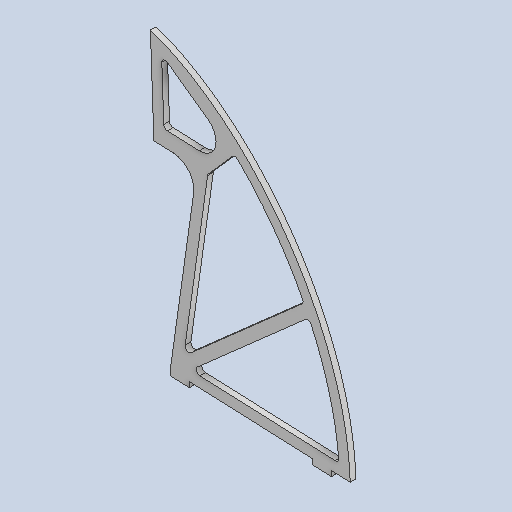
# Autodesk Inventor part: aux_nose_side
Saved by Autodesk Inventor 2022 (Build 260153000, 153)
## iProperties
Created: 2021-04-25
Part Number: aux_nose_side
Material: Generic
Document SubType Name: Modeling
Designer: kardo
Density: 1 g/cm^3
Appearance: Default
Mass: 3.39885 g
Surface Area: 48.7816 cm^2
Volume: 3.39885 cm^3
Author: kardo
Autodesk Inventor part; units mm, degrees
ref_plane "YZ Plane" through (0, 0, 0) normal (1, 0, 0) x (0, 1, 0)
ref_plane "XZ Plane" through (0, 0, 0) normal (0, 1, 0) x (-1, 0, 0)
ref_plane "XY Plane" through (0, 0, 0) normal (0, 0, 1) x (1, 0, 0)
derived "frame_outline.ipt"
sketch "aux_nose_side" plane through (81, 0, 28.1718) normal (0.0377663, 0.0348746, -0.9986779) x (0, 0.9993908, 0.0348995)
  line L0 (128.7776, 3.0021) -> (235.4965, 2.9535)
  line L1 (128.6834, 74.4231) -> (128.7776, 3.0021)
  line L2 (128.9392, -119.5453) -> (128.6076, 131.935)
  spline S0 degree 3 poles (128.6824, 75.2231) (178.453, 75.2888) (227.2802, 39.4794) (237.1445, 0) knots 0 0 0 0 1 1 1 1
  spline S1 degree 3 poles (128.6834, 74.4231) (132.6879, 74.4284) (140.6866, 73.9709) (150.5583, 72.3128) (160.2588, 69.9034) (167.8516, 67.4004) (177.0566, 63.6161) (184.1611, 60.0898) (192.6408, 55.123) (199.0732, 50.7282) (206.598, 44.7729) (212.1746, 39.6654) (218.5154, 32.9174) (223.0538, 27.2545) (227.9834, 19.911) (232.1324, 12.3358) (234.54, 6.0988) (235.4965, 2.9535) knots 0 0 0 0 0.081085 0.162171 0.202713 0.283799 0.324342 0.405427 0.44597 0.527055 0.567598 0.648683 0.689226 0.770311 0.810854 0.891939 0.973025 0.973025 0.973025 0.973025
  point P0 (-0.9832, -82.0055)
  point P1 (235.8467, 2.9533)
  point P2 (204.0556, 3.0021)
extrude "plate" add sketch "aux_nose_side" along normal blind 2
sketch "Sketch2" plane through (84, 128.6952, 32.7794) normal (-0.0377663, -0.0348746, 0.9986779) x (0.9992865, -0.0008625, 0.0377592)
  line L0 (71.4209, -0.1267) -> (0, 0) projected
  line L1 (71.4209, -0.1267) -> (0, 0) projected
  line L2 (57.1367, -0.1014) -> (57.1332, -2.1014)
  line L3 (57.1332, -2.1014) -> (64.2753, -2.1141)
  line L4 (64.2753, -2.1141) -> (64.2788, -0.1141)
  line L5 (3.571, -0.0063) -> (3.5675, -2.0063)
  line L6 (3.5675, -2.0063) -> (10.7096, -2.019)
  line L7 (10.7096, -2.019) -> (10.7131, -0.019)
  point P0 (-85.0668, -129.722)
  point P1 (64.2788, -0.1141)
  point P2 (57.1367, -0.1014)
  point P3 (10.7131, -0.019)
  point P4 (3.571, -0.0063)
  dimension "d28" = 71.421
  dimension "d29" = 7.1421
  dimension "d30" = 7.1421
  dimension "d31" = 2
  dimension "d32" = 3.5711
  dimension "d33" = 7.1421
  constraints: 12 end point, 4 perpendicular, 4 point on line, 2 parallel, 1 collinear
  measures "d28" distance of L0.start L0.end
  measures "d29" distance of L5.end L6.end
  measures "d30" distance of L2.end L3.end
  measures "d31" distance of L2.start L2.end
  measures "d32" distance of L5.start L0.end
  measures "d33" distance of L0.start L4.end
extrude "fins_break_plane" add sketch "Sketch2" against normal up to surface (2 mm away)
sketch "Sketch3" plane through (84, 128.6952, 32.7794) normal (-0.0377663, -0.0348746, 0.9986779) x (0.9992865, -0.0008625, 0.0377592)
  line L0 (10.7096, -2.019) -> (10.7131, -0.019) projected
  line L1 (57.1367, -0.1014) -> (57.1332, -2.1014) projected
  line L2 (0, 0) -> (0, 106.7189) projected
  spline S0 degree 3 poles (0, 106.7189) (3.1449, 105.7609) (9.3807, 103.3505) (16.954, 99.198) (24.2953, 94.2651) (29.9562, 89.7242) (36.7013, 83.3803) (41.8062, 77.8013) (47.758, 70.2738) (52.1499, 63.8394) (57.1129, 55.3575) (60.6359, 48.2513) (64.4161, 39.0446) (66.9157, 31.4506) (69.3206, 21.7491) (70.9741, 11.8766) (71.428, 3.8777) (71.4209, -0.1267) knots 0 0 0 0 0.083333 0.166667 0.208333 0.291667 0.333333 0.416667 0.458333 0.541667 0.583333 0.666667 0.708333 0.791667 0.833333 0.916667 1 1 1 1
  line L3 (3.571, -0.0063) -> (3.5675, -2.0063) projected
  line L4 (3.571, -0.0063) -> (14.7068, 62.4987)
  arc A0 (14.7068, 62.4987) -> (7.3534, 71.278) centre (7.3534, 63.8088) ccw
  line L5 (10.7131, -0.019) -> (10.3569, -2.0184) construction
  line L6 (3.5675, -2.0063) -> (10.7096, -2.019) projected
  line L7 (4, 77.278) -> (4, 101.0748)
  line L8 (8.3452, 3.9852) -> (67.3476, 3.8805)
  line L9 (71.4209, -0.1267) -> (64.2788, -0.1141) projected
  line L10 (7.3534, 71.278) -> (0, 71.278)
  line L11 (20.3339, 71.278) -> (8.3452, 3.9852)
  line L12 (3.571, -0.0063) -> (0, 0) projected
  line L13 (57.1367, -0.1014) -> (10.7131, -0.019) projected
  line L14 (8.9123, 7.1685) -> (55.7843, 48.9138)
  line L15 (11.3463, 3.9799) -> (57.5385, 45.1197)
  line L16 (17.3398, 77.278) -> (4, 77.278)
  arc A1 (17.3398, 77.278) -> (21.0802, 89.2615) centre (17.3398, 83.8535) ccw
  line L17 (21.0802, 89.2615) -> (4, 101.0748)
  line L18 (21.0802, 89.2615) -> (22.1137, 90.7559) construction
  line L19 (8.3452, 3.9852) -> (56.6752, 47.0291) construction
  line L20 (22.2644, 79.4962) -> (17.3398, 83.8535) construction
  line L21 (22.2644, 79.4962) -> (25.2601, 76.8456) construction
  line L22 (56.6752, 47.0291) -> (67.3476, 3.8805) construction
  line L23 (20.3339, 71.278) -> (30.952, 83.2785)
  line L24 (56.6752, 47.0291) -> (30.952, 83.2785) construction
  line L25 (0, 62.4987) -> (14.7068, 62.4987) construction
  line L26 (7.3534, 71.278) -> (7.3534, 62.4987) construction
  line L27 (0, 71.278) -> (0, 73.2783)
  line L28 (0, 73.2783) -> (0.0343, 75.278)
  line L29 (0.0343, 75.278) -> (0, 77.278)
  line L30 (0, 77.278) -> (4, 77.278)
  spline S1 degree 5 poles (4, 101.0748) (10.439, 98.5043) (16.5509, 95.1144) (22.262, 91.1174) (34.4968, 80.8283) (44.6435, 68.432) (49.7053, 60.9368) (58.1785, 45.5925) (63.8074, 29.0036) (65.8171, 20.7435) (67.0242, 12.3289) (67.3477, 3.8805) knots 0 0 0 0 0 0 0.284299 0.284299 0.284299 0.653322 0.653322 0.653322 1 1 1 1 1 1
  point P0 (-85.0668, -129.722)
  point P1 (64.2788, -0.1141)
  dimension "d41" = 4
  dimension "d12" = 106.7189
  dimension "d14" = 4
  dimension "d15" = 4
  dimension "d18" = 170
  dimension "d25" = 4
  dimension "d35" = 4
  dimension "d38" = 5
  dimension "d39" = 6
  dimension "d40" = 4
  dimension "d50" = 2
  constraints: 46 end point, 10 point on line, 5 parallel, 5 perpendicular, 5 point on circle, 4 tangent, 2 centre point, 2 collinear, 2 equal length, 1 midpoint, 1 vertical, 12 other
  measures "d12" distance of L2.start L2.end
  measures "d14" distance of the line from the sketch origin of L8
  measures "d15" distance between parallel lines of L2 L7
  measures "d18" angle of L5 L0
  measures "d25" distance between parallel lines of L14 L15
  measures "d35" distance between parallel lines of L4 L11
  measures "d39" distance between parallel lines of L10 L16
  measures "d40" distance of L20.start L21.end
  measures "d50" distance of L27.end L28.end
extrude "Extrusion4" cut sketch "Sketch3" against normal through all contours L2 L10 A0 L4 L12 | L7 L17 A1 L16 | L15 S1 L8
sketch "Sketch4" plane through (127.8536, 187.3715, 36.4868) normal (-0.0377663, -0.0348746, 0.9986779) x (0.9992857, -0.002636, 0.0376972)
  line L0 (-32.4682, -54.8278) -> (13.6509, -13.606) projected
  line L1 (-29.2116, 3.697) -> (-40.2363, -58.8278) projected
  arc A0 (-26.6048, 18.4808) -> (-22.8856, 30.471) centre (-26.6164, 25.0564) ccw projected
  line L2 (-34.9079, -51.6434) -> (11.89, -9.815)
  line L3 (-13.0033, 24.5055) -> (-23.6001, 12.4862)
  line L4 (-23.6001, 12.4862) -> (-34.9079, -51.6434)
  arc A1 (-26.6048, 18.4808) -> (-22.8856, 30.471) centre (-26.6164, 25.0564) ccw projected
  line L5 (-18.6837, 18.0625) -> (-26.6164, 25.0564) construction
  line L6 (-43.9339, 12.4501) -> (-36.5805, 12.4631) projected
  arc A2 (11.89, -9.815) -> (-13.0033, 24.5055) centre (-95.4946, -61.5148) ccw
  point P0 (-128.6438, -188.7006)
  point P1 (-21.6841, 20.7078)
  point P2 (0.9818, 8.4611)
  dimension "d44" = 4
  dimension "d45" = 4
  dimension "d46" = 4
  constraints: 8 end point, 4 point on circle, 3 point on line, 2 parallel, 1 centre point, 1 perpendicular, 8 other
  measures "d44" distance between parallel lines of L0 L2
  measures "d45" distance between parallel lines of L1 L4
  measures "d46" distance from line of point (-21.684, 20.708) L3
extrude "Extrusion5" cut sketch "Sketch4" against normal through all
fillet "Fillet2" radius 1.3333 9 edges at (92.9404, 135.8866, 32.3673) (87.9997, 205.9576, 34.6274) (104.3246, 199.9471, 35.0348) (95.3742, 132.6978, 32.3479) (87.9889, 229.7399, 35.4574) (114.9297, 211.9312, 35.8544) (141.5146, 173.7727, 35.5272) (139.76, 177.566, 35.5933) (151.3356, 132.5501, 34.459)
equation "\"d1\" = bulkhead_thickness"
equation "\"d29\" = 0.1 * d28"
equation "\"d30\" = 0.1 * d28"
equation "\"d32\" = 0.5 * d29"
equation "\"d33\" = d30"
equation "\"d14\" = inset"
equation "\"d15\" = inset"
equation "\"d25\" = inset"
equation "\"d35\" = inset"
equation "\"d39\" = 3 * bulkhead_thickness"
equation "\"d40\" = inset"
equation "\"bulkhead_thickness\" = 2"
equation "\"inset\" = 4"
body "Solid1"
